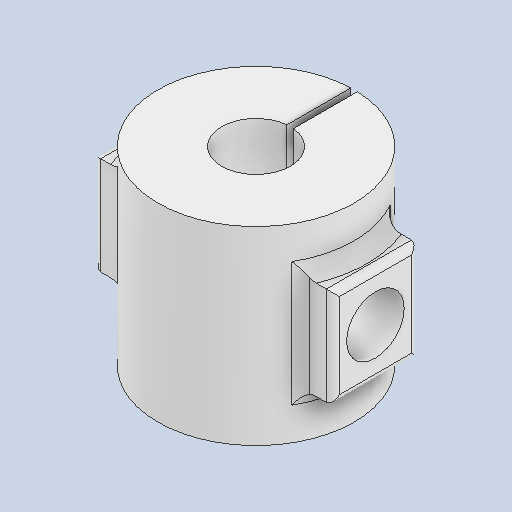
# Autodesk Inventor part: Space
Saved by Autodesk Inventor 2023 (Build 270158030, 158C)
## iProperties
Created: 2022-10-01
Part Number: Space
Material: ABS Plastic
Document SubType Name: Modeling
Designer: cjj5381
Density: 1.06 g/cm^3
Appearance: Smooth - White
Author: cjj5381
Autodesk Inventor part; units mm, degrees
ref_plane "YZ Plane" through (0, 0, 0) normal (1, 0, 0) x (0, 1, 0)
ref_plane "XZ Plane" through (0, 0, 0) normal (0, 1, 0) x (-1, 0, 0)
sketch "Sketch1" plane through (0, 0, 0) normal (0, 1, 0) x (-1, 0, 0)
  arc A0 (0.5, -14.9917) -> (-0.5, -14.9917) centre (0, 0) ccw
  arc A1 (0.5, -5.2261) -> (-0.5, -5.2261) centre (0, 0) ccw
  line L0 (-0.5, -5.2261) -> (-0.5, -14.9917)
  line L1 (0.5, -14.9917) -> (0.5, -5.2261)
  line L2 (0, 0) -> (0, -14.3069)
  dimension "d0" = 30
  dimension "d1" = 10.5
  dimension "d2" = 1
  constraints: 6 end point, 4 point on circle, 2 centre point, 2 coincident, 2 vertical, 1 parallel, 1 symmetric about line
  measures "d0" diameter of A0
  measures "d1" diameter of A1
  measures "d2" distance between parallel lines of L0 L1
extrude "Extrusion1" add sketch "Sketch1" along normal mid plane 29
ref_plane "Work Plane2" through (-15, 0, 0) normal (1, 0, 0) x (0, 0, -1)
sketch "Sketch3" plane through (-15, 0, 0) normal (1, 0, 0) x (0, 0, -1)
  line L0 (14.9917, -14.5) -> (5.2261, -14.5) projected
  line L1 (14.9917, 14.5) -> (14.9917, -14.5) projected
  point P0 (0, 0)
  point P1 (10.9917, -7)
  dimension "d6" = 7.5
  dimension "d7" = 4
  measures "d6" distance from line of L0 point (10.992, -7)
  measures "d7" distance from line of L1 point (10.992, -7)
hole "Hole1" at (-15, -7, -10.9917) direction (1, 0, 0) diameter 2.8 end through all counterbore diameter 6 counterbore depth 9
mirror "Mirror1" about plane through (0, 0, 0) normal (0, 1, 0) of "Hole1"
sketch "Sketch5" plane through (0, 0, 0) normal (0, 1, 0) x (-1, 0, 0)
  arc A0 (0.5, -14.9917) -> (-0.5, -14.9917) centre (0, 0) ccw projected
  line L0 (13.5185, 6.5) -> (18.25, 6.5)
  line L1 (18.25, 6.5) -> (18.25, -6.5)
  line L2 (18.25, -6.5) -> (13.5185, -6.5)
  line L3 (0, 0) -> (15.3886, 0)
  line L4 (0, 0) -> (0, -14.2024)
  arc A1 (13.5185, -6.5) -> (13.5185, 6.5) centre (0, 0) ccw
  line L5 (-13.5185, 6.5) -> (-18.25, 6.5)
  line L6 (-18.25, 6.5) -> (-18.25, -6.5)
  line L7 (-18.25, -6.5) -> (-13.5185, -6.5)
  arc A2 (-13.5185, 6.5) -> (-13.5185, -6.5) centre (0, 0) ccw
  arc A3 (0.5, -5.2261) -> (-0.5, -5.2261) centre (0, 0) ccw construction
  line L8 (5.25, 0) -> (5.25, -22.9648) construction
  point P0 (-15.3886, 0)
  dimension "d23" = 13
  dimension "d36" = 13
  constraints: 18 end point, 7 point on circle, 5 symmetric about line, 2 centre point, 2 horizontal, 2 perpendicular, 2 vertical, 1 concentric, 1 point on line, 1 tangent, 2 other
  measures "d23" distance of L0.end L1.end
  measures "d36" distance between parallel lines of L1 L8
extrude "Extrusion2" add sketch "Sketch5" along normal mid plane 15
sketch "Sketch6" plane through (-18.25, -7.5, 6.5) normal (-1, 0, 0) x (0, 0, 1)
  point P0 (-6.5, 7.5)
  point P1 (-6.5, 7.5)
  constraints: 1 coincident
hole "Hole3" at (-18.25, 0, 0) direction (1, 0, 0) diameter 8.8 end through all
fillet "Fillet1" radius 2 8 edges at (-13.5185, 0, -6.5) (-15, 7.5, 0) (-13.5185, 0, 6.5) (-15, -7.5, 0) (13.5185, 0, 6.5) (15, -7.5, 0) (13.5185, 0, -6.5) (15, 7.5, 0)
fillet "Fillet2" radius 1 8 edges at (18.25, 0, 6.5) (18.25, 7.5, 0) (18.25, 0, -6.5) (18.25, -7.5, 0) (-18.25, 0, 6.5) (-18.25, 7.5, 0) (-18.25, 0, -6.5) (-18.25, -7.5, 0)
body "Solid1"
